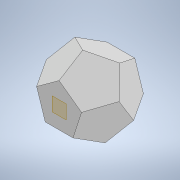
# Autodesk Inventor part: dodecahedron
Saved by Autodesk Inventor 2020.2 (Build 242310000, 310)
## iProperties
Created: 2020-01-17
Part Number: dodecahedron
Material: Generic
Document SubType Name: Modeling
Designer: Bardo91
Density: 1 g/cm^3
Appearance: Default
Author: Bardo91
Autodesk Inventor part; units mm, degrees
ref_plane "YZ Plane" through (0, 0, 0) normal (1, 0, 0) x (0, 1, 0)
ref_plane "XZ Plane" through (0, 0, 0) normal (0, 1, 0) x (-1, 0, 0)
ref_plane "Work Plane1" through (0, 0, 44.5407) normal (0, 0, 1) x (1, 0, 0)
sketch "Sketch2" plane through (0, 0, 44.5407) normal (0, 0, 1) x (1, 0, 0)
  line L0 (0, 34.026) -> (32.3607, 10.5146)
  line L1 (32.3607, 10.5146) -> (20, -27.5276)
  line L2 (20, -27.5276) -> (-20, -27.5276)
  line L3 (-20, -27.5276) -> (-32.3607, 10.5146)
  line L4 (-32.3607, 10.5146) -> (0, 34.026)
  point P0 (0, 0)
  point P1 (0, 0)
  dimension "d2" = 40
  constraints: 10 end point, 1 coincident, 11 other
  measures "d2" distance of L1.end L2.end
loft "Loft1" add profiles "Sketch2" section 2 point at (0, 0, 0)
mirror "Mirror1" about plane through (32.3607, 10.5146, 44.5407) normal (0.809017, -0.2628656, -0.5257311) of "Loft1"
mirror "Mirror2" about plane through (20, -27.5276, 44.5407) normal (0, -0.8506508, -0.5257311) of "Loft1"
mirror "Mirror3" about plane through (-20, -27.5276, 44.5407) normal (-0.809017, -0.2628656, -0.5257311) of "Loft1"
mirror "Mirror4" about plane through (-32.3607, 10.5146, 44.5407) normal (-0.5, 0.688191, -0.5257311) of "Loft1"
mirror "Mirror5" about plane through (0, 34.026, 44.5407) normal (0.5, 0.688191, -0.5257311) of "Loft1"
mirror "Mirror6" about plane through (-52.3607, -17.013, -10.5146) normal (0.309017, -0.4253254, -0.8506508) of "Loft1", "Mirror3"
mirror "Mirror7" about plane through (-52.3607, 17.013, 10.5146) normal (0, 0.5257311, -0.8506508) of "Loft1", "Mirror3"
mirror "Mirror8" about plane through (52.3607, -17.013, -10.5146) normal (0, 0.5257311, -0.8506508) of "Loft1", "Mirror1"
mirror "Mirror9" about plane through (20, 27.5276, -44.5407) normal (-0.809017, -0.2628656, -0.5257311) of "Loft1", "Mirror1", "Mirror8"
body "Solid1"
